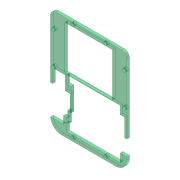
# Autodesk Inventor part: beagle_spacer_top
Saved by Autodesk Inventor 2014 (Build 180170000, 170)
## iProperties
Created: 2013-06-20
Part Number: beagle_spacer_top
Document SubType Name: Modeling
Designer: Administrator
Density: 1 g/cm^3
Mass: 10.2288 g
Surface Area: 93.7196 cm^2
Volume: 10.2288 cm^3
Material: Generic
Appearance: Clear - Green 1
Author: Administrator
Autodesk Inventor part; units mm, degrees
ref_plane "YZ Plane" through (0, 0, 0) normal (1, 0, 0) x (0, 1, 0)
ref_plane "XZ Plane" through (0, 0, 0) normal (0, 1, 0) x (-1, 0, 0)
ref_plane "XY Plane" through (0, 0, 0) normal (0, 0, 1) x (1, 0, 0)
sketch "Sketch1" plane through (0, 0, 0) normal (0, 0, 1) x (1, 0, 0)
  line L0 (9.8795, 48.1994) -> (9.8795, -53.4006)
  line L1 (16.2295, 54.5494) -> (92.4295, 54.5494)
  line L2 (98.7795, 48.1994) -> (98.7795, -53.4006)
  line L3 (22.5795, -66.1006) -> (86.0795, -66.1006)
  arc A0 (9.8795, -53.4006) -> (22.5795, -66.1006) centre (22.5795, -53.4006) ccw
  arc A1 (16.2295, 54.5494) -> (9.8795, 48.1994) centre (16.2295, 48.1994) ccw
  arc A2 (98.7795, 48.1994) -> (92.4295, 54.5494) centre (92.4295, 48.1994) ccw
  arc A3 (86.0795, -66.1006) -> (98.7795, -53.4006) centre (86.0795, -53.4006) ccw
  point P0 (0, 0)
  dimension "d0" = 12.7
  dimension "d1" = 6.35
  dimension "d2" = 120.65
  dimension "d3" = 88.9
  constraints: 8 end point, 8 point on circle, 8 tangent, 4 centre point, 2 equal radius, 1 horizontal, 1 vertical
  measures "d0" radius of A0
  measures "d1" radius of A1
  measures "d2" distance between parallel lines of L3 L1
  measures "d3" distance between parallel lines of L2 L0
extrude "Extrusion1" add sketch "Sketch1" along normal blind 3.175
sketch "Sketch2" plane through (0, 0, 3.175) normal (0, 0, 1) x (1, 0, 0)
  line L0 (9.8795, -53.4006) -> (9.8795, 48.1994) projected
  line L1 (98.7795, 48.1994) -> (98.7795, -53.4006) projected
  line L2 (16.2295, 54.5494) -> (92.4295, 54.5494) projected
  line L3 (26.6435, 49.4694) -> (82.0155, 49.4694)
  line L4 (82.0155, 49.4694) -> (82.0155, -1.3306)
  line L5 (82.0155, -1.3306) -> (26.6435, -1.3306)
  line L6 (26.6435, -1.3306) -> (26.6435, 49.4694)
  point P0 (0, 0)
  dimension "d13" = 16.764
  dimension "d14" = 16.764
  dimension "d15" = 5.08
  dimension "d16" = 55.88
  constraints: 8 end point
  measures "d13" distance between parallel lines of L0 L6
  measures "d14" distance between parallel lines of L1 L4
  measures "d15" distance between parallel lines of L2 L3
  measures "d16" distance between parallel lines of L5 L2
extrude "Extrusion2" cut sketch "Sketch2" against normal through all
sketch "Sketch3" plane through (0, 0, 3.175) normal (0, 0, 1) x (1, 0, 0)
  line L0 (9.8795, -53.4006) -> (9.8795, 48.1994) projected
  line L1 (86.0795, -66.1006) -> (22.5795, -66.1006) projected
  line L2 (9.8795, -19.4408) -> (32.7395, -19.4408)
  line L3 (32.7395, -19.4408) -> (32.7395, -37.2208)
  line L4 (32.7395, -37.2208) -> (9.8795, -37.2208)
  point P0 (0, 0)
  dimension "d20" = 28.8798
  dimension "d21" = 46.6598
  dimension "d22" = 22.86
  constraints: 6 end point, 2 point on line
  measures "d20" distance between parallel lines of L4 L1
  measures "d21" distance between parallel lines of L1 L2
  measures "d22" distance between parallel lines of L3 L0
extrude "Extrusion3" cut sketch "Sketch3" against normal through all
sketch "Sketch4" plane through (0, 0, 3.175) normal (0, 0, 1) x (1, 0, 0)
  line L0 (9.8795, -53.4006) -> (9.8795, -37.2208) projected
  arc A0 (9.8795, -53.4006) -> (22.5795, -66.1006) centre (22.5795, -53.4006) ccw projected
  line L1 (86.0795, -66.1006) -> (22.5795, -66.1006) projected
  line L2 (24.8655, -43.5708) -> (24.8655, -54.1626)
  line L3 (24.8655, -43.5708) -> (9.8795, -43.5708)
  line L4 (24.8655, -54.1626) -> (9.9024, -54.1626)
  point P0 (0, 0)
  dimension "d26" = 22.5298
  dimension "d27" = 14.986
  dimension "d28" = 11.938
  constraints: 6 end point, 1 horizontal, 1 point on circle, 1 point on line, 1 vertical
  measures "d26" distance between parallel lines of L1 L3
  measures "d27" distance between parallel lines of L0 L2
  measures "d28" distance between parallel lines of L1 L4
extrude "Extrusion4" cut sketch "Sketch4" against normal through all
sketch "Sketch5" plane through (0, 0, 3.175) normal (0, 0, 1) x (1, 0, 0)
  line L0 (86.0795, -66.1006) -> (22.5795, -66.1006) projected
  line L1 (9.8795, -19.4408) -> (9.8795, 48.1994) projected
  line L2 (9.8795, -43.5708) -> (9.8795, -37.2208) projected
  line L3 (28.9295, -2.1688) -> (91.1595, -2.1688)
  line L4 (91.1595, -2.1688) -> (91.1595, -11.5668)
  line L5 (91.1595, -11.5668) -> (28.9295, -11.5668)
  line L6 (28.9295, -11.5668) -> (28.9295, -2.1688)
  line L7 (28.9295, -50.4288) -> (91.1595, -50.4288)
  line L8 (91.1595, -50.4288) -> (91.1595, -59.8268)
  line L9 (91.1595, -59.8268) -> (28.9295, -59.8268)
  line L10 (28.9295, -59.8268) -> (28.9295, -50.4288)
  point P0 (0, 0)
  dimension "d31" = 54.5338
  dimension "d32" = 9.398
  dimension "d33" = 62.23
  dimension "d34" = 19.05
  dimension "d35" = 19.05
  dimension "d36" = 6.2738
  constraints: 16 end point, 2 equal length
  measures "d31" distance between parallel lines of L0 L5
  measures "d32" distance between parallel lines of L3 L5
  measures "d33" distance of L4.end L5.end
  measures "d34" distance between parallel lines of L1 L6
  measures "d35" distance between parallel lines of L2 L10
  measures "d36" distance between parallel lines of L9 L0
extrude "Extrusion5" cut sketch "Sketch5" against normal through all
sketch "Sketch8" plane through (0, 0, 3.175) normal (0, 0, 1) x (1, 0, 0)
  line L0 (91.1595, -11.5668) -> (28.9295, -11.5668) projected
  line L1 (28.9295, -50.4288) -> (91.1595, -50.4288) projected
  line L2 (91.1595, -50.4288) -> (91.1595, -59.8268) projected
  line L3 (9.8795, -43.5708) -> (24.8655, -43.5708) projected
  line L4 (24.8655, -43.5708) -> (24.8655, -54.1626) projected
  line L5 (86.0795, -66.1006) -> (22.5795, -66.1006) projected
  line L6 (98.7795, 48.1994) -> (98.7795, -53.4006) projected
  line L7 (9.8795, -19.4408) -> (9.8795, 48.1994) projected
  line L8 (9.8795, -19.4408) -> (32.7395, -19.4408) projected
  line L9 (32.7395, -37.2208) -> (9.8795, -37.2208) projected
  line L10 (9.8795, -43.5708) -> (9.8795, -37.2208) projected
  line L11 (96.2395, -11.5668) -> (96.2395, -32.3948)
  line L12 (96.2395, -32.3948) -> (98.7795, -32.3948)
  line L13 (91.1595, -11.5668) -> (96.2395, -11.5668)
  line L14 (98.7795, -50.1748) -> (91.1595, -50.1748)
  line L15 (9.8795, -3.4388) -> (27.1515, -3.4388)
  line L16 (27.1515, -3.4388) -> (27.1515, -19.4408)
  line L17 (34.0095, -11.5668) -> (34.0095, -38.3638)
  line L18 (31.2155, -38.3638) -> (31.2155, -50.4288)
  line L19 (30.0725, -37.2208) -> (30.0725, -45.4758)
  line L20 (24.8655, -45.4758) -> (30.0725, -45.4758)
  line L21 (31.2155, -38.3638) -> (34.0095, -38.3638)
  line L22 (91.1595, -50.4288) -> (91.1595, -50.1748)
  line L23 (12.4195, -3.4388) -> (12.4195, -19.4408)
  point P0 (0, 0)
  dimension "d63" = 2.54
  dimension "d67" = 15.9258
  dimension "d68" = 16.002
  dimension "d69" = 17.272
  dimension "d70" = 24.13
  dimension "d71" = 21.336
  dimension "d72" = 1.143
  dimension "d73" = 1.143
  dimension "d76" = 17.78
  dimension "d78" = 2.54
  dimension "d79" = 1.905
  constraints: 26 end point, 11 point on line, 2 horizontal
  measures "d63" distance between parallel lines of L6 L11
  measures "d67" distance between parallel lines of L5 L14
  measures "d68" distance between parallel lines of L8 L15
  measures "d69" distance between parallel lines of L7 L16
  measures "d70" distance between parallel lines of L7 L17
  measures "d71" distance between parallel lines of L10 L18
  measures "d72" distance between parallel lines of L18 L19
  measures "d73" distance between parallel lines of L9 L21
  measures "d76" distance between parallel lines of L14 L12
  measures "d78" distance between parallel lines of L7 L23
  measures "d79" distance between parallel lines of L3 L20
extrude "Extrusion11" cut sketch "Sketch8" against normal through all contours L13 L11 L12 L6 L14 L22 L1 L18 L21 L17 L0 | L10 L9 L19 L20 L4 L3 | L23 L15 L16 L8
sketch "Sketch9" plane through (0, 0, 3.175) normal (0, 0, 1) x (1, 0, 0)
  line L0 (98.7795, 48.1994) -> (98.7795, -32.3948) projected
  line L1 (16.2295, 54.5494) -> (92.4295, 54.5494) projected
  line L2 (9.8795, -19.4408) -> (9.8795, 48.1994) projected
  line L3 (86.0795, -66.1006) -> (22.5795, -66.1006) projected
  line L4 (36.2694, 49.7107) -> (34.2897, 49.7107)
  line L5 (34.2897, 49.7107) -> (33.2998, 51.4252)
  line L6 (33.2998, 51.4252) -> (34.2897, 53.1397)
  line L7 (34.2897, 53.1397) -> (36.2694, 53.1397)
  line L8 (36.2694, 53.1397) -> (37.2593, 51.4252)
  line L9 (37.2593, 51.4252) -> (36.2694, 49.7107)
  line L10 (14.7182, 34.5095) -> (13.0037, 33.5197)
  line L11 (13.0037, 33.5197) -> (11.2892, 34.5095)
  line L12 (11.2892, 34.5095) -> (11.2892, 36.4893)
  line L13 (11.2892, 36.4893) -> (13.0037, 37.4791)
  line L14 (13.0037, 37.4791) -> (14.7182, 36.4893)
  line L15 (14.7182, 36.4893) -> (14.7182, 34.5095)
  line L16 (14.7182, -3.5905) -> (13.0037, -4.5803)
  line L17 (13.0037, -4.5803) -> (11.2892, -3.5905)
  line L18 (11.2892, -3.5905) -> (11.2892, -1.6107)
  line L19 (11.2892, -1.6107) -> (13.0037, -0.6209)
  line L20 (13.0037, -0.6209) -> (14.7182, -1.6107)
  line L21 (14.7182, -1.6107) -> (14.7182, -3.5905)
  line L22 (75.3593, 51.4252) -> (74.3694, 49.7107)
  line L23 (74.3694, 49.7107) -> (72.3897, 49.7107)
  line L24 (72.3897, 49.7107) -> (71.3998, 51.4252)
  line L25 (71.3998, 51.4252) -> (72.3897, 53.1397)
  line L26 (72.3897, 53.1397) -> (74.3694, 53.1397)
  line L27 (74.3694, 53.1397) -> (75.3593, 51.4252)
  line L28 (97.3698, 34.5095) -> (95.6553, 33.5197)
  line L29 (95.6553, 33.5197) -> (93.9408, 34.5095)
  line L30 (93.9408, 34.5095) -> (93.9408, 36.4893)
  line L31 (93.9408, 36.4893) -> (95.6553, 37.4791)
  line L32 (95.6553, 37.4791) -> (97.3698, 36.4893)
  line L33 (97.3698, 36.4893) -> (97.3698, 34.5095)
  line L34 (95.6553, -4.5803) -> (93.9408, -3.5905)
  line L35 (93.9408, -3.5905) -> (93.9408, -1.6107)
  line L36 (93.9408, -1.6107) -> (95.6553, -0.6209)
  line L37 (95.6553, -0.6209) -> (97.3698, -1.6107)
  line L38 (97.3698, -1.6107) -> (97.3698, -3.5905)
  line L39 (97.3698, -3.5905) -> (95.6553, -4.5803)
  line L40 (36.2694, -64.6909) -> (34.2897, -64.6909)
  line L41 (34.2897, -64.6909) -> (33.2998, -62.9764)
  line L42 (33.2998, -62.9764) -> (34.2897, -61.2619)
  line L43 (34.2897, -61.2619) -> (36.2694, -61.2619)
  line L44 (36.2694, -61.2619) -> (37.2593, -62.9764)
  line L45 (37.2593, -62.9764) -> (36.2694, -64.6909)
  line L46 (75.3593, -62.9764) -> (74.3694, -64.6909)
  line L47 (74.3694, -64.6909) -> (72.3897, -64.6909)
  line L48 (72.3897, -64.6909) -> (71.3998, -62.9764)
  line L49 (71.3998, -62.9764) -> (72.3897, -61.2619)
  line L50 (72.3897, -61.2619) -> (74.3694, -61.2619)
  line L51 (74.3694, -61.2619) -> (75.3593, -62.9764)
  point P0 (0, 0)
  point P1 (35.2795, 51.4252)
  point P2 (13.0037, 35.4994)
  point P3 (13.0037, -2.6006)
  point P4 (73.3795, 51.4252)
  point P5 (95.6553, 35.4994)
  point P6 (95.6553, -2.6006)
  point P7 (35.2795, -62.9764)
  point P8 (73.3795, -62.9764)
  dimension "d80" = 3.1242
  dimension "d81" = 3.1242
  dimension "d82" = 38.1
  dimension "d83" = 3.429
  dimension "d84" = 19.05
  dimension "d85" = 25.4
  dimension "d86" = 38.1
  dimension "d87" = 3.1242
  dimension "d88" = 3.1242
  constraints: 96 end point, 7 equal length, 4 horizontal, 4 horizontal alignment, 4 vertical, 4 vertical alignment, 104 other
  measures "d80" distance from line of L2 point (13.004, 35.499)
  measures "d81" distance from line of L1 point (35.28, 51.425)
  measures "d82" distance of point (13.004, 35.499) point (13.004, -2.601)
  measures "d83" distance between parallel lines of L4 L7
  measures "d84" distance from line of L1 point (13.004, 35.499)
  measures "d85" distance from line of L2 point (35.28, 51.425)
  measures "d86" distance of point (73.38, 51.425) point (35.28, 51.425)
  measures "d87" distance from line of L3 point (35.28, -62.976)
  measures "d88" distance from line of L0 point (95.655, 35.499)
extrude "Extrusion12" cut sketch "Sketch9" against normal through all
sketch "Sketch10" plane through (0, 0, 0) normal (0, 0, -1) x (-1, 0, 0)
  line L0 (-14.7182, -3.4388) -> (-14.7182, -1.6107) projected
  line L1 (-14.7182, -1.6107) -> (-13.0037, -0.6209) projected
  line L2 (-13.0037, -0.6209) -> (-11.2892, -1.6107) projected
  line L3 (-11.2892, -1.6107) -> (-11.2892, -3.5905) projected
  line L4 (-11.2892, -3.5905) -> (-12.4195, -4.243) projected
  line L5 (-12.4195, -4.243) -> (-12.4195, -19.4408) projected
  line L6 (-12.4195, -19.4408) -> (-9.8795, -19.4408) projected
  line L7 (-9.8795, 48.1994) -> (-9.8795, -19.4408) projected
  arc A0 (-9.8795, 48.1994) -> (-16.2295, 54.5494) centre (-16.2295, 48.1994) ccw projected
  line L8 (-92.4295, 54.5494) -> (-16.2295, 54.5494) projected
  arc A1 (-92.4295, 54.5494) -> (-98.7795, 48.1994) centre (-92.4295, 48.1994) ccw projected
  line L9 (-98.7795, -32.3948) -> (-98.7795, 48.1994) projected
  line L10 (-98.7795, -32.3948) -> (-96.2395, -32.3948) projected
  line L11 (-96.2395, -32.3948) -> (-96.2395, -11.5668) projected
  line L12 (-96.2395, -11.5668) -> (-91.1595, -11.5668) projected
  line L13 (-91.1595, -11.5668) -> (-91.1595, -2.1688) projected
  line L14 (-91.1595, -2.1688) -> (-28.9295, -2.1688) projected
  line L15 (-28.9295, -2.1688) -> (-28.9295, -11.5668) projected
  line L16 (-28.9295, -11.5668) -> (-34.0095, -11.5668) projected
  line L17 (-34.0095, -11.5668) -> (-34.0095, -38.3638) projected
  line L18 (-34.0095, -38.3638) -> (-31.2155, -38.3638) projected
  line L19 (-31.2155, -38.3638) -> (-31.2155, -50.4288) projected
  line L20 (-31.2155, -50.4288) -> (-28.9295, -50.4288) projected
  line L21 (-28.9295, -50.4288) -> (-28.9295, -59.8268) projected
  line L22 (-28.9295, -59.8268) -> (-91.1595, -59.8268) projected
  line L23 (-91.1595, -59.8268) -> (-91.1595, -50.1748) projected
  line L24 (-91.1595, -50.1748) -> (-98.7795, -50.1748) projected
  line L25 (-98.7795, -53.4006) -> (-98.7795, -50.1748) projected
  arc A2 (-98.7795, -53.4006) -> (-86.0795, -66.1006) centre (-86.0795, -53.4006) ccw projected
  line L26 (-22.5795, -66.1006) -> (-86.0795, -66.1006) projected
  arc A3 (-22.5795, -66.1006) -> (-9.9024, -54.1626) centre (-22.5795, -53.4006) ccw projected
  line L27 (-9.9024, -54.1626) -> (-24.8655, -54.1626) projected
  line L28 (-24.8655, -54.1626) -> (-24.8655, -45.4758) projected
  line L29 (-24.8655, -45.4758) -> (-30.0725, -45.4758) projected
  line L30 (-30.0725, -45.4758) -> (-30.0725, -37.2208) projected
  line L31 (-30.0725, -37.2208) -> (-32.7395, -37.2208) projected
  line L32 (-32.7395, -37.2208) -> (-32.7395, -19.4408) projected
  line L33 (-32.7395, -19.4408) -> (-27.1515, -19.4408) projected
  line L34 (-27.1515, -19.4408) -> (-27.1515, -3.4388) projected
  line L35 (-27.1515, -3.4388) -> (-14.7182, -3.4388) projected
  line L36 (-26.6435, 49.4694) -> (-26.6435, -1.3306) projected
  line L37 (-26.6435, -1.3306) -> (-82.0155, -1.3306) projected
  line L38 (-82.0155, -1.3306) -> (-82.0155, 49.4694) projected
  line L39 (-82.0155, 49.4694) -> (-26.6435, 49.4694) projected
  line L40 (-97.3698, 34.5095) -> (-97.3698, 36.4893) projected
  line L41 (-97.3698, 36.4893) -> (-95.6553, 37.4791) projected
  line L42 (-95.6553, 37.4791) -> (-93.9408, 36.4893) projected
  line L43 (-93.9408, 36.4893) -> (-93.9408, 34.5095) projected
  line L44 (-93.9408, 34.5095) -> (-95.6553, 33.5197) projected
  line L45 (-95.6553, 33.5197) -> (-97.3698, 34.5095) projected
  line L46 (-14.7182, 34.5095) -> (-14.7182, 36.4893) projected
  line L47 (-14.7182, 36.4893) -> (-13.0037, 37.4791) projected
  line L48 (-13.0037, 37.4791) -> (-11.2892, 36.4893) projected
  line L49 (-11.2892, 36.4893) -> (-11.2892, 34.5095) projected
  line L50 (-11.2892, 34.5095) -> (-13.0037, 33.5197) projected
  line L51 (-13.0037, 33.5197) -> (-14.7182, 34.5095) projected
  line L52 (-36.2694, -64.6909) -> (-37.2593, -62.9764) projected
  line L53 (-37.2593, -62.9764) -> (-36.2694, -61.2619) projected
  line L54 (-36.2694, -61.2619) -> (-34.2897, -61.2619) projected
  line L55 (-34.2897, -61.2619) -> (-33.2998, -62.9764) projected
  line L56 (-33.2998, -62.9764) -> (-34.2897, -64.6909) projected
  line L57 (-34.2897, -64.6909) -> (-36.2694, -64.6909) projected
  line L58 (-75.3593, 51.4252) -> (-74.3694, 53.1397) projected
  line L59 (-74.3694, 53.1397) -> (-72.3897, 53.1397) projected
  line L60 (-72.3897, 53.1397) -> (-71.3998, 51.4252) projected
  line L61 (-71.3998, 51.4252) -> (-72.3897, 49.7107) projected
  line L62 (-72.3897, 49.7107) -> (-74.3694, 49.7107) projected
  line L63 (-74.3694, 49.7107) -> (-75.3593, 51.4252) projected
  line L64 (-75.3593, -62.9764) -> (-74.3694, -61.2619) projected
  line L65 (-74.3694, -61.2619) -> (-72.3897, -61.2619) projected
  line L66 (-72.3897, -61.2619) -> (-71.3998, -62.9764) projected
  line L67 (-71.3998, -62.9764) -> (-72.3897, -64.6909) projected
  line L68 (-72.3897, -64.6909) -> (-74.3694, -64.6909) projected
  line L69 (-74.3694, -64.6909) -> (-75.3593, -62.9764) projected
  line L70 (-95.6553, -4.5803) -> (-97.3698, -3.5905) projected
  line L71 (-97.3698, -3.5905) -> (-97.3698, -1.6107) projected
  line L72 (-97.3698, -1.6107) -> (-95.6553, -0.6209) projected
  line L73 (-95.6553, -0.6209) -> (-93.9408, -1.6107) projected
  line L74 (-93.9408, -1.6107) -> (-93.9408, -3.5905) projected
  line L75 (-93.9408, -3.5905) -> (-95.6553, -4.5803) projected
  line L76 (-36.2694, 49.7107) -> (-37.2593, 51.4252) projected
  line L77 (-37.2593, 51.4252) -> (-36.2694, 53.1397) projected
  line L78 (-36.2694, 53.1397) -> (-34.2897, 53.1397) projected
  line L79 (-34.2897, 53.1397) -> (-33.2998, 51.4252) projected
  line L80 (-33.2998, 51.4252) -> (-34.2897, 49.7107) projected
  line L81 (-34.2897, 49.7107) -> (-36.2694, 49.7107) projected
  point P0 (0, 0)
  dimension "d91" = 16.764
  dimension "d92" = 72.136
  dimension "d93" = 115.57
  dimension "d94" = 64.77
  measures "d91" distance between parallel lines of L9 L38
  measures "d92" distance between parallel lines of L9 L36
  measures "d93" distance between parallel lines of L26 L39
  measures "d94" distance between parallel lines of L26 L37
equation "\"d14\" = d13"
equation "\"d35\" = d34"
equation "\"d73\" = d72"
body "Solid1"
